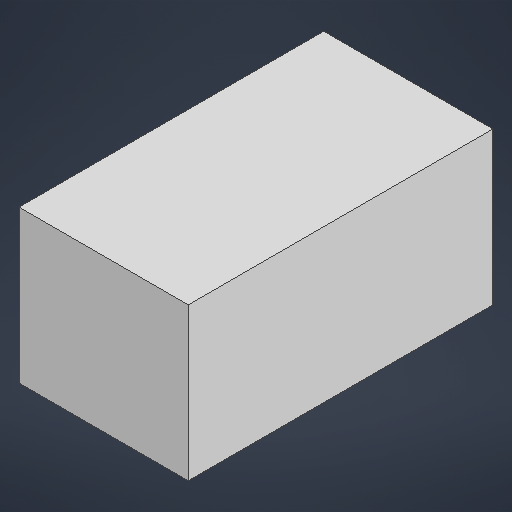
# Autodesk Inventor part: Controller Handle
Saved by Autodesk Inventor 2026.2 (Build 302298010, 298A)
## iProperties
Created: 2026-03-08
Part Number: Controller Handle
Material: Generic
Document SubType Name: Modeling
Designer: barbe
Density: 1 g/cm^3
Appearance: Default
Author: barbe
Autodesk Inventor part; units mm, degrees
ref_plane "YZ Plane" through (0, 0, 0) normal (1, 0, 0) x (0, 1, 0)
ref_plane "XZ Plane" through (0, 0, 0) normal (0, 1, 0) x (-1, 0, 0)
ref_plane "XY Plane" through (0, 0, 0) normal (0, 0, 1) x (1, 0, 0)
sketch "Sketch1" plane through (0, 0, 0) normal (1, 0, 0) x (0, 1, 0)
  line L0 (-11.43, 22.86) -> (11.43, 22.86)
  line L1 (11.43, 22.86) -> (11.43, -22.86)
  line L2 (11.43, -22.86) -> (-11.43, -22.86)
  line L3 (-11.43, -22.86) -> (-11.43, 22.86)
  line L4 (-11.43, 22.86) -> (11.43, -22.86) construction
  line L5 (11.43, 22.86) -> (-11.43, -22.86) construction
  point P0 (0, 0)
  dimension "d0" = 22.86
  dimension "d1" = 45.72
  constraints: 12 end point, 2 midpoint, 2 parallel, 1 horizontal, 1 perpendicular
  measures "d0" distance of L1.end L2.end
  measures "d1" distance of L0.end L1.end
extrude "Extrusion1" add sketch "Sketch1" along normal blind 25.4
sketch "Sketch2" plane through (0, 0, 0) normal (-1, 0, 0) x (0, 0, 1)
  line L0 (-10.795, 8.89) -> (10.795, 8.89)
  line L1 (10.795, 8.89) -> (10.795, -8.89)
  line L2 (10.795, -8.89) -> (-10.795, -8.89)
  line L3 (-10.795, -8.89) -> (-10.795, 8.89)
  line L4 (-10.795, 8.89) -> (10.795, -8.89) construction
  line L5 (10.795, 8.89) -> (-10.795, -8.89) construction
  point P0 (0, 0)
  dimension "d4" = 21.59
  dimension "d5" = 17.78
  constraints: 12 end point, 2 midpoint, 2 parallel, 1 horizontal, 1 perpendicular
  measures "d4" distance of L1.end L2.end
  measures "d5" distance of L0.end L1.end
extrude "Extrusion2" cut sketch "Sketch2" against normal blind 12.7
sketch "Sketch3" plane through (0, 0, 0) normal (-1, 0, 0) x (0, 0, 1)
  line L0 (-10.795, -8.89) -> (-10.795, 8.89) projected
  point P0 (0, 0)
  point P1 (-17.145, 0.8313)
  dimension "d8" = 6.35
  measures "d8" distance from line of L0 point (-17.145, 0.831)
hole "Hole1" at (0, 0.8313, -17.145) direction (1, 0, 0) diameter 4 depth 8
thread "Thread1" size "M4x0.7" class "6H" standard "ANSI Metric M Profile" full length
mirror "Mirror1" about plane through (0, 0, 0) normal (0, 0, 1) of "Hole1"
thread "Thread2" size "M4x0.7" class "6H" standard "ANSI Metric M Profile" length 8.001
body "Solid1"
